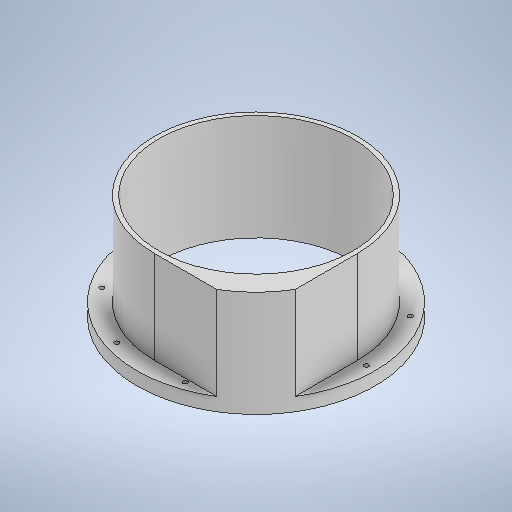
# Autodesk Inventor part: Cylinder Housing
Saved by Autodesk Inventor 2025 (Build 290162000, 162)
## iProperties
Created: 2025-06-17
Part Number: Cylinder Housing
Material: Generic
Document SubType Name: Modeling
Designer: mumin
Density: 1 g/cm^3
Appearance: Default
Author: mumin
Autodesk Inventor part; units mm, degrees
ref_plane "YZ Plane" through (0, 0, 0) normal (1, 0, 0) x (0, 1, 0)
ref_plane "XZ Plane" through (0, 0, 0) normal (0, 1, 0) x (-1, 0, 0)
ref_plane "XY Plane" through (0, 0, 0) normal (0, 0, 1) x (1, 0, 0)
sketch "Sketch1" plane through (0, 0, 0) normal (0, 1, 0) x (-1, 0, 0)
  circle A0 centre (0, 0) radius 110
  circle A1 centre (0, 0) radius 135
  dimension "d0" = 220
  dimension "d1" = 270
  constraints: 2 centre point, 2 coincident
  measures "d0" diameter of A0
  measures "d1" diameter of A1
extrude "Extrusion1" add sketch "Sketch1" along normal blind 15
sketch "Sketch5" plane through (0, 15, 0) normal (0, 1, 0) x (1, 0, 0)
  line L0 (-189, 0) -> (189, 0) projected
  point P0 (0, 0)
  point P1 (-125, 0)
  dimension "d23" = 125
  constraints: 1 point on line
  measures "d23" distance of point (0, 0) point (-125, 0)
hole "Hole2" at (-125, 15, 0) direction (0, -1, 0) diameter 5.2 end through all
pattern_circular "Circular Pattern1" count 10 over 360 about axis through (0, -10, 0) along (0, 1, 0) of "Hole2"
sketch "Sketch6" plane through (0, 0, 0) normal (0, 1, 0) x (-1, 0, 0)
  circle A0 centre (0, 0) radius 110 projected
  circle A1 centre (0, 0) radius 135 projected
  circle A2 centre (0, 0) radius 115
  line L0 (0, 115) -> (-115, 115)
  line L1 (-115, 115) -> (-115, 0)
  point P0 (-70.7107, 115)
  point P1 (-115, 70.7107)
  dimension "d27" = 230
  constraints: 4 end point, 2 point on circle, 2 tangent, 1 centre point, 1 coincident, 1 horizontal
  measures "d27" diameter of A2
extrude "Extrusion4" add sketch "Sketch6" along normal blind 120 contours L0 A2 L1 A1 | A2 picked at (-94.2438, 86.8114)
body "Solid1"
